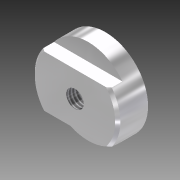
# Autodesk Inventor part: Auumulator Cap 1764
Saved by Autodesk Inventor 2011 (Build 150239000, 239)
## iProperties
Created: 2010-01-18
Part Number: Auumulator Cap 1764
Document SubType Name: Modeling
Designer: cmcfadden
Density: 1 g/cm^3
Author: cmcfadden
Autodesk Inventor part; units mm, degrees
ref_plane "YZ Plane" through (0, 0, 0) normal (1, 0, 0) x (0, 1, 0)
ref_plane "XZ Plane" through (0, 0, 0) normal (0, 1, 0) x (-1, 0, 0)
ref_plane "XY Plane" through (0, 0, 0) normal (0, 0, 1) x (1, 0, 0)
sketch "Sketch1" plane through (0, 0, 0) normal (0, 0, 1) x (1, 0, 0)
  circle A0 centre (-14.977, 17.3579) radius 26.4414
  point P0 (0, 0)
  dimension "d0" = 52.8828
  constraints: 1 centre point
  measures "d0" diameter of A0
extrude "Extrusion1" add sketch "Sketch1" along normal blind 18.7198
chamfer "Chamfer1" distance 1.5875 angle 45 1 edges at (-41.4184, 17.3579, 18.7198)
sketch "Sketch2" plane through (-14.977, 17.3579, 18.7198) normal (0, 0, 1) x (1, 0, 0)
  circle A0 centre (0, 0) radius 24.8539 projected
  circle A1 centre (0, 0) radius 26.4414 projected
  line L0 (-21.1455, -15.875) -> (21.1455, -15.875)
  line L1 (-21.1455, 15.875) -> (21.1455, 15.875)
  arc A2 (21.1455, 15.875) -> (-21.1455, 15.875) centre (0, 0) ccw
  arc A3 (-21.1455, -15.875) -> (21.1455, -15.875) centre (0, 0) ccw
  point P0 (14.977, -17.3579)
  dimension "d6" = 31.75
  dimension "d7" = 15.875
  constraints: 8 point on circle, 4 end point, 2 centre point, 2 concentric, 1 horizontal
  measures "d6" distance between parallel lines of L0 L1
  measures "d7" distance from line of A0.centre L1
extrude "Extrusion2" cut sketch "Sketch2" against normal blind 8.128 contours L1 A0 | A0 L1 A1 | L0 A1 A0 | A0 L0
sketch "Sketch3" plane through (0, 0, 18.7198) normal (0, 0, 1) x (1, 0, 0)
  arc A0 (-34.1003, 33.2329) -> (-34.1003, 1.4829) centre (-14.977, 17.3579) ccw projected
  circle A1 centre (-14.977, 17.3579) radius 5.3975
  point P0 (0, 0)
  dimension "d10" = 10.795
  constraints: 1 centre point, 1 coincident
  measures "d10" diameter of A1
extrude "Extrusion3" cut sketch "Sketch3" against normal through all
thread "Thread1" size "9/16-12 UNC" class "2B" standard "ANSI Unified Screw Threads" full length
body "Solid1"
